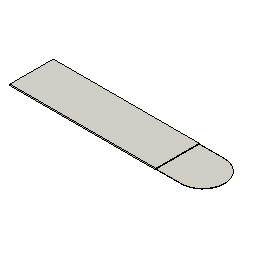
ESPing_Assembled (Autodesk Fusion 360 archive; units mm, degrees)
design "Command Strip - N/Velcro"
Autodesk Fusion 360 part; units mm, degrees
sketch "Sketch1" plane through (0, 0, 0) normal (0, 0, 1) x (1, 0, 0)
  line L0 (0, 7.875) -> (62.125, 7.875)
  arc A0 (62.125, -7.875) -> (62.125, 7.875) centre (62.125, 0) ccw
  line L1 (62.125, -7.875) -> (0, -7.875)
  line L2 (0, -7.875) -> (0, 7.875)
  line L3 (53, 7.875) -> (53, -7.875)
  dimension "d1" = 15.75
  dimension "d2" = 70
  dimension "d3" = 53
  constraint horizontal L0
  constraint tangent L0 A0
  constraint parallel L0 L1
  constraint perpendicular L0 L2
  constraint tangent A0 L1
  constraint midpoint L2 origin
  constraint coincident L0 L3.start
  constraint coincident L1 L3.end
  constraint perpendicular L1 L3
  measures "d1" distance of L0.start L1.end
  measures "d3" distance of L2 L3
extrude "Extrude1" add sketch "Sketch1" along normal mid plane 0.5 contours L0 L1 L2 L3
extrude "Extrude2" add sketch "Sketch1" along normal mid plane 0.14 contours L0 A0 L1 L3

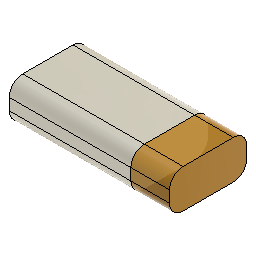
design "102040 LiPo Battery"
Autodesk Fusion 360 part; units mm, degrees
box "BoxPrimitive1" add length 20 width 41.5 height 10 placed x (0, 1, 0) y (-1, 0, 0) z (0, 0, 1) at (41.5, 0, 0)
ref_plane "WorkPlane1" through (31.5, 10, 5) normal (1, 0, 0) x (0, 0, -1)
sketch "Sketch4" plane through (0, 0, 0) normal (-1, 0, 0) x (0, -1, 0)
  line L0 (-20, 10) -> (-20, 0) construction
  line L1 (-20, 0) -> (0, 0) construction
  line L2 (0, 0) -> (0, 10) construction
  line L3 (0, 10) -> (-20, 10) construction
  arc A0 (-16.5, 10) -> (-20, 6.5) centre (-16.5, 6.5) ccw
  line L4 (-16.5, 10) -> (-10, 10) construction
  line L5 (-20, 5) -> (-20, 6.5) construction
  line L6 (-20, 5) -> (0, 5) construction
  line L7 (-10, 10) -> (-10, 0) construction
  line L8 (-20, 6.5) -> (-20, 10)
  line L9 (-16.5, 10) -> (-20, 10)
  line L10 (0, 6.5) -> (0, 10)
  arc A1 (0, 6.5) -> (-3.5, 10) centre (-3.5, 6.5) ccw
  line L11 (-3.5, 10) -> (0, 10)
  line L12 (-20, 3.5) -> (-20, 0)
  arc A2 (-20, 3.5) -> (-16.5, 0) centre (-16.5, 3.5) ccw
  line L13 (-16.5, 0) -> (-20, 0)
  line L14 (0, 3.5) -> (0, 0)
  arc A3 (-3.5, 0) -> (0, 3.5) centre (-3.5, 3.5) ccw
  line L15 (-3.5, 0) -> (0, 0)
  point P0 (-10, 10)
  point P1 (-10, 10)
  point P2 (0, 5)
  point P3 (0, 5)
  point P4 (-20, 5)
  point P5 (-20, 5)
  dimension "d12" = 6.5
  constraint coincident L0 A0.end
  constraint midpoint L3 P1
  constraint coincident P1 P0
  constraint midpoint L2 P3
  constraint coincident P3 P2
  constraint midpoint L0 P5
  constraint coincident P5 P4
  constraint coincident L3 A0.start
  constraint tangent A0 L4
  constraint tangent A0 L5
  constraint midpoint L1 L7.end
  constraint coincident L0.start L3.end
  constraint symmetric A0.end L7 L10.start
  constraint symmetric A0.start L7 A1.end
  constraint symmetric A0 L7 A1
  constraint symmetric L7 L0.start L2.end
  constraint symmetric A0.end L6 L12.start
  constraint symmetric A0.start L6 A2.end
  constraint symmetric A0 L6 A2
  constraint symmetric L6 L0.start L0.end
  constraint symmetric L6 L10.start L14.start
  constraint symmetric L6 L2.end L1.end
  constraint symmetric L6 A1.end A3.start
  constraint symmetric L6 A1 A3
  measures "d12" distance of A0.start P1
extrude "Extrude1" cut sketch "Sketch4" against normal up to surface (41.5 mm away)
split_face "SplitFace1" 8 faces at (13.8333, 7.8333, 10) (27.6667, 0, 4.5) (13.8333, 7.8333, 0) (27.6667, 20, 4.5) (27.6667, 0.4689, 8.25) (27.6667, 2.6748, 0.0987) (27.6667, 17.8008, 9.7493) (27.6667, 17.6447, 0.1925) by plane through (31.5, 10, 5) normal (1, 0, 0)

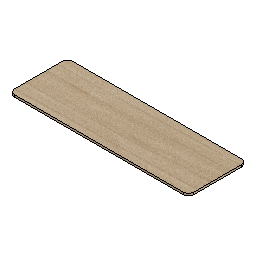
design "ESPing_Bottom_Liner"
Autodesk Fusion 360 part; units mm, degrees
sketch "Sketch1" plane through (0, 0, 0.1137) normal (0, 0, -1) x (1, 0, 0)
  line L0 (72.5484, -22.1397) -> (-5.3516, -22.1397) construction
  line L1 (-5.3516, -22.1397) -> (-5.3516, -0.3397) construction
  line L2 (-5.3516, -0.3397) -> (72.5484, -0.3397) construction
  line L3 (72.5484, -0.3397) -> (72.5484, -22.1397) construction
  arc A0 (75.1, -0.2881) -> (72.6, 2.2119) centre (72.6, -0.2881) ccw construction
  line L4 (72.6, 2.2119) -> (-5.4031, 2.2119) construction
  arc A1 (-5.4031, 2.2119) -> (-7.9031, -0.2881) centre (-5.4031, -0.2881) ccw construction
  line L5 (-7.9031, -0.2881) -> (-7.9031, -22.1912) construction
  arc A2 (-7.9031, -22.1912) -> (-5.4031, -24.6912) centre (-5.4031, -22.1912) ccw construction
  line L6 (-5.4031, -24.6912) -> (72.6, -24.6912) construction
  arc A3 (72.6, -24.6912) -> (75.1, -22.1912) centre (72.6, -22.1912) ccw construction
  line L7 (75.1, -22.1912) -> (75.1, -0.2881) construction
  line L8 (-3.1516, -0.5397) -> (-3.1516, -21.9397) construction
  line L9 (-3.1516, -21.9397) -> (-1.1516, -21.9397) construction
  line L10 (-1.1516, -21.9397) -> (-1.1516, -0.5397) construction
  line L11 (-1.1516, -0.5397) -> (-3.1516, -0.5397) construction
  line L12 (1.8484, -11.9397) -> (2.3484, -11.9397) construction
  line L13 (2.3484, -11.9397) -> (2.3484, -21.9397) construction
  line L14 (2.3484, -21.9397) -> (32.8484, -21.9397) construction
  line L15 (32.8484, -21.9397) -> (32.8484, -11.9397) construction
  line L16 (32.8484, -11.9397) -> (33.3484, -11.9397) construction
  line L17 (33.3484, -11.9397) -> (33.3484, -21.9397) construction
  line L18 (33.3484, -21.9397) -> (72.3484, -21.9397) construction
  line L19 (72.3484, -21.9397) -> (72.3484, -0.5397) construction
  line L20 (72.3484, -0.5397) -> (-0.1516, -0.5397) construction
  line L21 (-0.1516, -0.5397) -> (-0.1516, -21.9397) construction
  line L22 (-0.1516, -21.9397) -> (1.8484, -21.9397) construction
  line L23 (1.8484, -21.9397) -> (1.8484, -11.9397) construction
  circle A4 centre (45.2984, -13.4098) radius 1.8
  line L24 (-4.6016, -0.3397) -> (-3.9016, -0.3397)
  line L25 (-3.1516, -1.0897) -> (-3.1516, -21.3897)
  line L26 (-3.9016, -22.1397) -> (-4.6016, -22.1397)
  line L27 (-5.3516, -21.3897) -> (-5.3516, -1.0897)
  line L28 (-5.4031, 2.2119) -> (72.6, 2.2119)
  arc A5 (75.1, -0.2881) -> (72.6, 2.2119) centre (72.6, -0.2881) ccw
  line L29 (75.1, -0.2881) -> (75.1, -22.1912)
  arc A6 (72.6, -24.6912) -> (75.1, -22.1912) centre (72.6, -22.1912) ccw
  line L30 (72.6, -24.6912) -> (-5.4031, -24.6912)
  arc A7 (-7.9031, -22.1912) -> (-5.4031, -24.6912) centre (-5.4031, -22.1912) ccw
  line L31 (-7.9031, -22.1912) -> (-7.9031, -0.2881)
  arc A8 (-5.4031, 2.2119) -> (-7.9031, -0.2881) centre (-5.4031, -0.2881) ccw
  arc A9 (-4.6016, -0.3397) -> (-5.3516, -1.0897) centre (-4.6016, -1.0897) ccw
  arc A10 (-3.1516, -1.0897) -> (-3.9016, -0.3397) centre (-3.9016, -1.0897) ccw
  arc A11 (-3.9016, -22.1397) -> (-3.1516, -21.3897) centre (-3.9016, -21.3897) ccw
  arc A12 (-5.3516, -21.3897) -> (-4.6016, -22.1397) centre (-4.6016, -21.3897) ccw
  dimension "d551" = 0.75
  constraint horizontal L24
  constraint vertical L25
  constraint horizontal L26
  constraint vertical L27
  constraint collinear L8 L25
  constraint coincident L4.end A1.start
  constraint coincident A0.end L4.start
  constraint coincident A0.start L7.end
  constraint tangent L4 A5
  constraint coincident A3.end L7.start
  constraint coincident L6.end A3.start
  constraint tangent L7 A6
  constraint coincident A2.end L6.start
  constraint coincident L5.end A2.start
  constraint tangent L30 A7
  constraint coincident A1.end L5.start
  constraint tangent L31 A8
  constraint tangent L24 A9
  constraint tangent L27 A9
  constraint tangent L24 A10
  constraint tangent L25 A10
  constraint equal A9 A10
  constraint tangent L25 A11
  constraint tangent L26 A11
  constraint equal A9 A11
  constraint tangent L26 A12
  constraint tangent L27 A12
  constraint equal A9 A12
  constraint collinear L1 L27
  constraint collinear L0 L26
  constraint collinear L2 L24
  measures "d551" radius of A9
extrude "Extrude1" add sketch "Sketch1" along normal blind 1
sketch "Bottom Laser Cut Template" plane through (0, 0, -0.8863) normal (0, 0, -1) x (1, 0, 0)
  circle A0 centre (45.2984, -13.4098) radius 1.8
  arc A1 (-4.6016, -0.3397) -> (-5.3516, -1.0897) centre (-4.6016, -1.0897) ccw
  line L0 (-4.6016, -0.3397) -> (-3.9016, -0.3397)
  arc A2 (-3.1516, -1.0897) -> (-3.9016, -0.3397) centre (-3.9016, -1.0897) ccw
  line L1 (-3.1516, -1.0897) -> (-3.1516, -21.3897)
  arc A3 (-3.9016, -22.1397) -> (-3.1516, -21.3897) centre (-3.9016, -21.3897) ccw
  line L2 (-3.9016, -22.1397) -> (-4.6016, -22.1397)
  arc A4 (-5.3516, -21.3897) -> (-4.6016, -22.1397) centre (-4.6016, -21.3897) ccw
  line L3 (-5.3516, -21.3897) -> (-5.3516, -1.0897)
  arc A5 (75.1, -0.2881) -> (72.6, 2.2119) centre (72.6, -0.2881) ccw
  line L4 (72.6, 2.2119) -> (-5.4031, 2.2119)
  arc A6 (-5.4031, 2.2119) -> (-7.9031, -0.2881) centre (-5.4031, -0.2881) ccw
  line L5 (-7.9031, -0.2881) -> (-7.9031, -22.1912)
  arc A7 (-7.9031, -22.1912) -> (-5.4031, -24.6912) centre (-5.4031, -22.1912) ccw
  line L6 (-5.4031, -24.6912) -> (72.6, -24.6912)
  arc A8 (72.6, -24.6912) -> (75.1, -22.1912) centre (72.6, -22.1912) ccw
  line L7 (75.1, -22.1912) -> (75.1, -0.2881)
delete_face "DeleteFace1" 1 faces at (44.0416, 14.6984, -0.5529)
delete_face "DeleteFace2" 1 faces at (-5.0366, 22.0006, -0.5529)
delete_face "DeleteFace3" 1 faces at (-5.1444, 0.5721, -0.5529)
delete_face "DeleteFace4" 1 faces at (-3.7247, 0.3608, -0.5529)
delete_face "DeleteFace5" 1 faces at (-3.1651, 21.5316, -0.5529)
delete_face "DeleteFace6" 1 faces at (-3.1516, 7.6063, -0.2196)
split "Split1" [rolled back]
delete_body "RemoveBody1" bodies 2
fillet "Fillet1" [rolled back] radius 2.5
